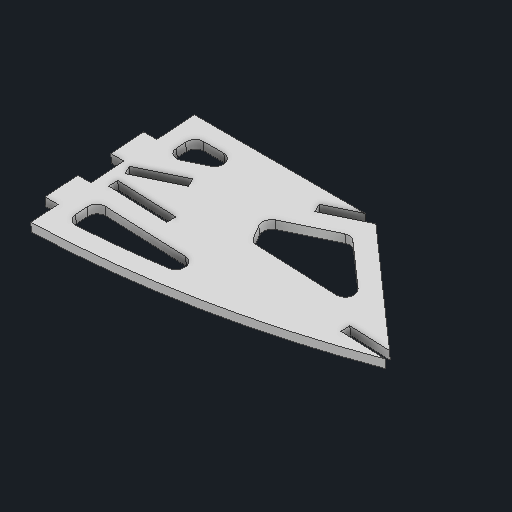
# Autodesk Inventor part: sponson_break
Saved by Autodesk Inventor 2022.2 (Build 262287010, 287A)
## iProperties
Created: 2022-03-21
Part Number: sponson_break
Material: Generic
Document SubType Name: Modeling
Designer: kardo
Density: 1 g/cm^3
Appearance: Default
Author: kardo
Autodesk Inventor part; units mm, degrees
ref_plane "YZ Plane" through (0, 0, 0) normal (1, 0, 0) x (0, 1, 0)
ref_plane "XZ Plane" through (0, 0, 0) normal (0, 1, 0) x (-1, 0, 0)
ref_plane "XY Plane" through (0, 0, 0) normal (0, 0, 1) x (1, 0, 0)
derived "parameters_frame.ipt"
derived "surface_body.ipt"
sketch "sk_rail_sponson_tunnel" plane through (81.12, 0, 0) normal (1, 0, 0) x (0, 1, 0)
  line L0 (0, 0) -> (135.09, 9.4464)
  line L1 (125.2485, 150.1861) -> (152.4642, -239.0164) construction
  spline S0 degree 2 poles (135.09, 9.4464) (188.144, 13.1563) (237, 36.448) knots 0 0 0 1 1 1
sketch "sk_rail_sponson_bottom" plane through (126.048, 0, 0) normal (0.4037383, -0.0638184, 0.9126459) x (-0.1841621, 0.9714748, 0.1494022)
  line L0 (132.6478, -27.2597) -> (0, 0)
  line L1 (373.4222, -76.7399) -> (-490.1731, 100.7327) construction
  line L2 (179.8623, 202.4893) -> (98.6127, -192.8771) construction
  spline S0 degree 2 poles (132.6478, -27.2597) (191.4823, -39.3504) (243.959, 0) knots 0 0 0 1 1 1
  point P0 (23.2133, 112.9576)
sketch "sk_rail_sponson_side" plane through (81.12, 237, 36.448) normal (0.0378267, 0.0348745, -0.9986756) x (0.3011979, -0.9533106, -0.0218819)
  line L0 (248.6073, 0) -> (121.4703, -40.1899)
  spline S0 degree 2 poles (121.4703, -40.1899) (54.6944, -61.2988) (0, 0) knots 0 0 0 1 1 1
  point P0 (202.299, 150.0824)
ref_plane "plane_sponson_break" through (0, 135.09, 9.4464) normal (0, 0.9975641, 0.0697565) x (-1, 0, 0)
sketch "sk_section_sponson_break" plane through (0, 135.09, 9.4464) normal (0, 0.9975641, 0.0697565) x (-1, 0, 0)
  line L0 (-276.9076, -66.575) -> (63.0269, 83.4396) construction
  line L1 (-81.12, -263.4566) -> (-81.12, 154.4936) construction
  arc A0 (-81.12, 40.0762) -> (-156, 26.279) centre (-76.0371, -197.602) ccw construction
  arc A1 (-54.6, 54.2675) -> (-156, 30.9325) centre (-53.2768, -183.4615) ccw construction
  spline S0 degree 2 poles (-54.6, 54.2675) (-107.2974, 54.2675) (-156, 30.9325) knots 0 0 0 1 1 1
  spline S1 degree 2 poles (-156, 26.279) (-119.9166, 39.1668) (-81.12, 40.0762) knots 0 0 0 1 1 1
  point P0 (0, 0)
derived "stencil_frame.ipt"
sketch "sk_joint_locations" plane through (81.12, 0, 0) normal (1, 0, 0) x (0, 1, 0)
  line L0 (0, 0) -> (135.09, 9.4464) construction
  line L1 (30.81, 28.832) -> (94.8, 28.832) construction
  arc A0 (30.81, 28.832) -> (9.48, 28.4869) centre (30.81, -630.4631) ccw construction
  line L2 (-254.1001, 19.9549) -> (9.48, 28.4869) construction
  line L3 (-363, 18.496) -> (-275.8801, 19.4795) construction
  arc A1 (-275.8801, 19.4795) -> (-254.1001, 19.9549) centre (-287.5515, 1053.3708) ccw construction
  line L4 (25.1322, 1581.9163) -> (267.6663, -1886.4825) construction
  line L5 (-242.0001, 1541.8302) -> (-242.0001, -1877.3857) construction
  line L6 (-120.9999, 1541.8302) -> (-120.9999, -1877.3857) construction
  line L7 (-363, 1541.8302) -> (-363, -1877.3857) construction
  line L8 (0, 1541.8302) -> (0, -1877.3857) construction
  line L9 (450.0665, 43.8884) -> (-613.9211, 6.7332) construction
  line L10 (-677.4829, -27.4989) -> (501.7293, 54.9597) construction
  line L11 (187.7215, 30.7247) -> (187.4423, 38.7198) construction
  line L12 (195.4031, 37.5588) -> (195.9625, 29.5588) construction
  line L13 (0, 3.808) -> (134.9306, 11.7256) construction
  line L14 (-242.0001, 45.8501) -> (-242.0001, 20.3465) construction
  line L15 (-363, 37.4293) -> (-363, 18.496) construction
  line L16 (-120.9999, 51.0063) -> (-120.9999, 24.2633) construction
  line L17 (0, 52.89) -> (0, 28.18) construction
  line L18 (132.2944, 49.425) -> (132.8217, 41.8851) construction
  line L19 (133.3489, 34.3453) -> (132.8217, 41.8851) construction
  line L20 (133.3489, 34.3453) -> (133.8761, 26.8054) construction
  line L21 (133.8761, 26.8054) -> (134.4034, 19.2655) construction
  line L22 (134.4034, 19.2655) -> (134.9306, 11.7256) construction
  line L23 (0, 3.808) -> (0, 0) construction
  spline S0 degree 4 poles (-363, 37.4293) (-272.3626, 45.1427) (-181.5879, 49.7528) (-90.8131, 52.89) (0, 52.89) knots 0 0 0 0 0 1 1 1 1 1
  spline S1 degree 3 poles (0, 52.89) (86.3106, 52.89) (181.3207, 49.5034) (237, 36.448) knots 0 0 0 0 1 1 1 1
  spline S2 degree 2 poles (135.09, 9.4464) (188.144, 13.1563) (237, 36.448) knots 0 0 0 1 1 1
  line L24 (94.8, 37.536) -> (94.8, 28.832) construction
  line L25 (94.8, 35.548) -> (94.8, 30.82) construction
  point P0 (187.5819, 34.7223)
  point P1 (195.6828, 33.5588)
  point P2 (134.9575, 11.3411)
  point P3 (-363, 27.9627)
  point P4 (-242.0001, 33.0983)
  point P5 (-120.9999, 37.6348)
  point P6 (0, 40.535)
  point P7 (94.8, 33.184)
sketch "sk_spanner_joints_locations" plane through (0, 135.09, 9.4464) normal (0, 0.9975641, 0.0697565) x (-1, 0, 0)
  line L0 (266.3539, 10.2816) -> (-340.3092, 33.2601) construction
  line L1 (-958.4738, -367.3533) -> (724.0529, 375.1534) construction
  line L2 (-86.9102, 23.6621) -> (-85.7837, 17.7688) construction
  line L3 (-86.9102, 23.6621) -> (-73.574, 23.157) construction
  line L4 (-85.7837, 17.7688) -> (-73.574, 23.157) construction
  point P0 (0, 0)
  point P1 (-126.048, 0)
  point P2 (-156, 26.279)
  point P3 (-142.182, 25.7557)
  point P4 (-100.7281, 24.1855)
  point P5 (-95.8498, 13.3266)
  point P6 (-115.9819, 4.4422)
sketch "sk_sponson_break_base" plane through (0, 135.09, 9.4464) normal (0, 0.9975641, 0.0697565) x (-1, 0, 0)
  spline S0 degree 2 poles (-156, 26.279) (-119.9166, 39.1668) (-81.12, 40.0762) knots 0 0 0 1 1 1 construction
  line L0 (-156, 26.279) -> (-126.048, 0) construction
  line L1 (-126.048, 0) -> (-81.12, 0) construction
  line L2 (-81.12, 32.5179) -> (-81.12, 24.9597)
  line L3 (-81.12, 24.9597) -> (-84.12, 24.9597)
  line L4 (-81.12, 32.5179) -> (-84.12, 32.5179)
  line L5 (-84.12, 32.5179) -> (-84.12, 38.7871)
  line L6 (-84.12, 24.9597) -> (-84.12, 17.4014)
  line L7 (-84.12, 17.4014) -> (-81.12, 17.4014)
  line L8 (-81.12, 17.4014) -> (-81.12, 9.8431)
  line L9 (-81.12, 9.8431) -> (-84.12, 9.8431)
  line L10 (-84.12, 9.8431) -> (-84.12, 1.2)
  line L11 (-153.6672, 25.8287) -> (-125.5962, 1.2)
  line L12 (-125.5962, 1.2) -> (-84.12, 1.2)
  spline S1 degree 5 poles (-84.12, 38.7871) (-98.3131, 38.2809) (-112.4697, 36.756) (-126.4909, 34.1573) (-140.2522, 30.4911) (-153.6672, 25.8287) knots 0 0 0 0 0 0 1 1 1 1 1 1
  point P0 (0, 0)
  point P1 (-156, 26.279)
  dimension "d4" = 1.2
  dimension "d3" = 3
  constraints: 26 end point, 6 parallel, 4 perpendicular, 1 vertical, 4 other
  measures "d3" distance from line of L7.end L6
extrude "thicken" add sketch "sk_sponson_break_base" against normal blind 2
sketch "sk_spanner_joints" plane through (0, 135.09, 9.4464) normal (0, 0.9975641, 0.0697565) x (-1, 0, 0)
  line L0 (-156, 26.279) -> (-142.182, 25.7557)
  line L1 (-142.182, 25.7557) -> (-142.2577, 23.7571)
  line L2 (-142.2577, 23.7571) -> (-156.0757, 24.2805)
  line L3 (-156.0757, 24.2805) -> (-156, 26.279)
  line L4 (-100.7281, 24.1855) -> (-100.8038, 22.1869)
  line L5 (-100.8038, 22.1869) -> (-86.9859, 21.6636)
  line L6 (-86.9859, 21.6636) -> (-86.9102, 23.6621)
  line L7 (-100.7281, 24.1855) -> (-86.9102, 23.6621)
  line L8 (-95.8498, 13.3266) -> (-96.6572, 15.1564)
  line L9 (-96.6572, 15.1564) -> (-86.5912, 19.5986)
  line L10 (-86.5912, 19.5986) -> (-85.7837, 17.7688)
  line L11 (-85.7837, 17.7688) -> (-95.8498, 13.3266)
  line L12 (-126.048, 0) -> (-115.9819, 4.4422)
  line L13 (-115.9819, 4.4422) -> (-116.7894, 6.272)
  line L14 (-116.7894, 6.272) -> (-126.8555, 1.8297)
  line L15 (-126.8555, 1.8297) -> (-126.048, 0)
  point P0 (0, 0)
  dimension "d7" = 2
  constraints: 32 end point, 8 perpendicular, 7 equal length
  measures "d7" distance of L2.end L0.start
extrude "cut_spanner_joints" cut sketch "sk_spanner_joints" along normal through all both and the other way through all
sketch "sk_cut_weight" plane through (0, 135.09, 9.4464) normal (0, 0.9975641, 0.0697565) x (-1, 0, 0)
  spline S0 degree 3 poles (-84.12, 38.7871) (-88.1153, 38.6446) (-95.0685, 38.2268) (-102.9379, 37.4125) (-108.8071, 36.6575) (-112.7034, 36.0819) (-117.5533, 35.2723) (-121.4168, 34.5524) (-126.2258, 33.5623) (-130.0565, 32.6981) (-134.8246, 31.5276) (-138.6227, 30.519) (-143.3499, 29.168) (-148.0568, 27.7267) (-151.8007, 26.4774) (-153.6672, 25.8287) knots 0.026839 0.026839 0.026839 0.026839 0.182488 0.299224 0.338137 0.415961 0.454873 0.532698 0.57161 0.649434 0.688346 0.766171 0.805083 0.882907 0.960732 0.960732 0.960732 0.960732 construction
  line L0 (-153.6672, 25.8287) -> (-125.5962, 1.2) construction
  line L1 (-125.5962, 1.2) -> (-84.12, 1.2) construction
  line L2 (-86.9102, 23.6621) -> (-156, 26.279) construction
  line L3 (-85.7837, 17.7688) -> (-126.048, 0) construction
  line L4 (-82.313, 21.4866) -> (-151.7143, 24.1153) construction
  line L5 (-82.313, 21.4866) -> (-126.4952, 1.9887) construction
  line L6 (-84.12, 38.7871) -> (-84.12, 1.2) construction
  line L7 (-88.12, 34.6064) -> (-88.12, 27.7108)
  line L8 (-88.12, 27.7108) -> (-127.3693, 29.1975)
  line L9 (-104.8581, 1.2) -> (-117.0136, 22.8009) construction
  line L10 (-140.6074, 19.6917) -> (-114.712, 18.7109)
  line L11 (-111.4889, 12.9833) -> (-125.7754, 6.6786)
  line L12 (-125.7754, 6.6786) -> (-140.6074, 19.6917)
  line L13 (-114.712, 18.7109) -> (-111.4889, 12.9833)
  line L14 (-88.12, 12.3656) -> (-104.3573, 5.2)
  line L15 (-104.3573, 5.2) -> (-88.12, 5.2)
  line L16 (-88.12, 5.2) -> (-88.12, 12.3656)
  spline S1 degree 4 poles (-88.12, 34.6064) (-98.023, 34.0832) (-107.8987, 33.0167) (-117.6966, 31.3846) (-127.3693, 29.1974) knots 0 0 0 0 0 1 1 1 1 1
  point P0 (0, 0)
  dimension "d12" = 4
  dimension "d10" = 2
  dimension "d11" = 2
  dimension "d13" = 4
  dimension "d14" = 4
  dimension "d15" = 4
  dimension "d16" = 4
  dimension "d17" = 4
  dimension "d18" = 4
  dimension "d19" = 4
  dimension "d20" = 4
  constraints: 30 end point, 10 parallel, 4 point on line, 2 midpoint, 3 other
  measures "d10" distance between parallel lines of L2 L4
  measures "d11" distance between parallel lines of L3 L5
  measures "d13" distance between parallel lines of L2 L8
  measures "d14" distance between parallel lines of L6 L7
  measures "d15" distance between parallel lines of L0 L12
  measures "d16" distance between parallel lines of L4 L10
  measures "d17" distance between parallel lines of L5 L11
  measures "d18" distance between parallel lines of L1 L15
  measures "d19" distance between parallel lines of L6 L16
  measures "d20" distance between parallel lines of L3 L14
extrude "cut_weight" cut sketch "sk_cut_weight" along normal through all both and the other way through all
fillet "Fillet1" radius 2 10 edges at (104.3573, 133.7297, 14.564) (88.12, 133.2299, 21.7121) (88.12, 133.7297, 14.564) (125.7754, 133.6266, 16.039) (111.4889, 133.1868, 22.3283) (88.12, 132.1594, 37.02) (114.712, 132.7872, 28.0419) (140.6074, 132.7188, 29.0204) (127.3693, 132.0557, 38.503) (88.12, 131.6784, 43.8987)
equation "\"d4\" = shell_thickness"
equation "\"d3\" = stringer_thickness"
equation "\"d5\" = bulkhead_thickness"
equation "\"d7\" = bulkhead_thickness"
equation "\"d12\" = bulkhead_inset"
equation "\"d10\" = bulkhead_thickness"
equation "\"d11\" = bulkhead_thickness"
equation "\"d13\" = bulkhead_inset"
equation "\"d14\" = bulkhead_inset"
equation "\"d15\" = bulkhead_inset"
equation "\"d16\" = bulkhead_inset"
equation "\"d17\" = bulkhead_inset"
equation "\"d18\" = bulkhead_inset"
equation "\"d19\" = bulkhead_inset"
equation "\"d20\" = bulkhead_inset"
equation "\"d23\" = 0.5 * bulkhead_inset"
equation "\"shell_thickness\" = 1.2"
equation "\"stringer_thickness\" = 3"
equation "\"bulkhead_thickness\" = 2"
equation "\"bulkhead_inset\" = 4"
body "Solid1"
